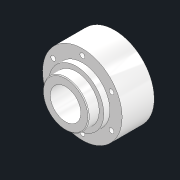
# Autodesk Inventor part: base6
Saved by Autodesk Inventor 2022 (Build 260153000, 153)
## iProperties
Created: 2021-09-16
Part Number: base6
Material: ABS プラスチック
Document SubType Name: Modeling
Designer: Yuta Kage
Density: 1.06 g/cm^3
Appearance: 滑らか - 白
Author: Yuta Kage
Autodesk Inventor part; units mm, degrees
ref_plane "YZ Plane" through (0, 0, 0) normal (1, 0, 0) x (0, 1, 0)
ref_plane "XZ Plane" through (0, 0, 0) normal (0, 1, 0) x (-1, 0, 0)
ref_plane "XY Plane" through (0, 0, 0) normal (0, 0, 1) x (1, 0, 0)
sketch "スケッチ1" plane through (0, 0, 0) normal (1, 0, 0) x (0, 1, 0)
  line L0 (15, 0) -> (15, -7)
  line L1 (15, -7) -> (18, -7)
  line L2 (26, -32) -> (10, -32)
  line L3 (10, -32) -> (10, 0)
  line L4 (10, 0) -> (15, 0)
  line L5 (0, -38.4) -> (0, 6.4) projected
  line L6 (18, -7) -> (18, -11)
  line L7 (18, -11) -> (26, -11)
  line L8 (26, -11) -> (26, -32)
  point P0 (0, 0)
  dimension "d0" = 10
  dimension "d1" = 15
  dimension "d2" = 7
  dimension "d3" = 3
  dimension "d10" = 25
  dimension "d11" = 4
  dimension "d12" = 8
  constraints: 16 end point, 5 perpendicular, 2 vertical, 1 horizontal alignment
  measures "d0" distance from line of point (0, 0) L3
  measures "d1" distance from line of point (0, 0) L0
  measures "d2" distance of L0.start L0.end
  measures "d3" distance of L0.end L1.end
  measures "d10" distance between parallel lines of L2 L1
  measures "d11" distance of L1.end L6.end
  measures "d12" distance of L6.end L7.end
revolve "回転1" add sketch "スケッチ1" angle 360 about axis through (0, 0, -10) along (0, 0, 1)
chamfer "面取り1" distance 0.5 angle 45 1 edges at (0, -15, 0)
sketch "スケッチ2" plane through (0, 0, -11) normal (0, 0, 1) x (1, 0, 0)
  circle A0 centre (0, 0) radius 26 projected
  circle A1 centre (0, 0) radius 22
  point P0 (0, 22)
  point P1 (-19.0526, 11)
  point P2 (-19.0526, -11)
  point P3 (0, -22)
  point P4 (19.0526, -11)
  point P5 (19.0526, 11)
  dimension "d13" = 4
  dimension "d16" = 360
  constraints: 1 vertical alignment, 9 other
hole "穴1" at (0, 22, -11) at (-19.0526, 11, -11) at (-19.0526, -11, -11) at (0, -22, -11) at (19.0526, -11, -11) at (19.0526, 11, -11) direction (0, 0, -1) diameter 3.2 end through all clearance for "Socket Head Cap Screw" size "M3" standard "Ansi Metric M Profile"
